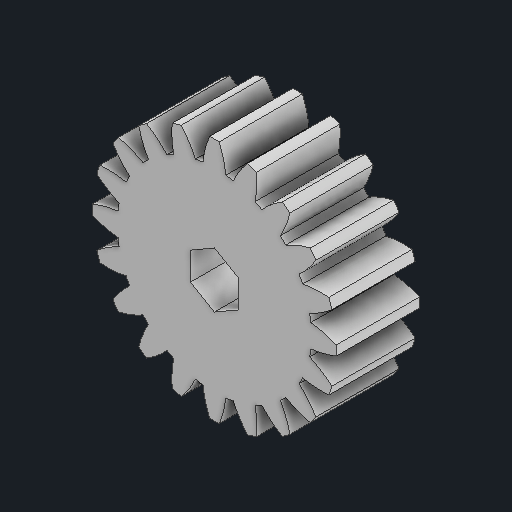
# Autodesk Inventor part: gear_wheel_base
Saved by Autodesk Inventor 2024 (Build 280153000, 153)
## iProperties
Created: 2023-06-19
Part Number: gear_wheel_base
Material: 일반
Document SubType Name: Modeling
Designer: 6gioc
Density: 1 g/cm^3
Appearance: 기본값
Author: 6gioc
Autodesk Inventor part; units mm, degrees
ref_plane "YZ Plane" through (0, 0, 0) normal (1, 0, 0) x (0, 1, 0)
ref_plane "XZ Plane" through (0, 0, 0) normal (0, 1, 0) x (-1, 0, 0)
ref_plane "XY Plane" through (0, 0, 0) normal (0, 0, 1) x (1, 0, 0)
sketch "스케치1" plane through (0, 0, 0) normal (0, 0, 1) x (1, 0, 0)
  circle A0 centre (0, 0) radius 22
  circle A1 centre (0, 0) radius 5
  line L0 (0, -5) -> (-4.3301, -2.5)
  line L1 (-4.3301, -2.5) -> (-4.3301, 2.5)
  line L2 (-4.3301, 2.5) -> (0, 5)
  line L3 (0, 5) -> (4.3301, 2.5)
  line L4 (4.3301, 2.5) -> (4.3301, -2.5)
  line L5 (4.3301, -2.5) -> (0, -5)
  dimension "d1" = 10
  dimension "d0" = 44
  constraints: 12 end point, 3 coincident, 1 centre point, 1 vertical alignment, 15 other
  measures "d0" diameter of A0
extrude "돌출1" add sketch "스케치1" along normal blind 15 contours A0 | A1 L4 | L3 A1 | A1 L5 | L2 A1 | A1 L0 | L1 A1
spur gear teeth "스퍼 기어1" teeth 20 pitch diameter 40 tip diameter 44 root diameter 35 face width 15 trims to tip circle yes start plane through (0, 0, 15) normal (0, 0, 1) x (1, 0, 0)
